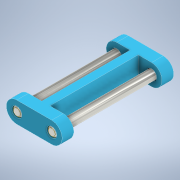
# Autodesk Inventor part: Lever
Saved by Autodesk Inventor 2021 (Build 250183000, 183)
## iProperties
Created: 2020-03-13
Part Number: Lever
Material: Generisch
Document SubType Name: Modeling
Designer: JochenAlt
Density: 1 g/cm^3
Appearance: Türkis
Author: JochenAlt
Autodesk Inventor part; units mm, degrees
ref_plane "YZ Plane" through (0, 0, 0) normal (1, 0, 0) x (0, 1, 0)
ref_plane "XZ Plane" through (0, 0, 0) normal (0, 1, 0) x (-1, 0, 0)
ref_plane "XY Plane" through (0, 0, 0) normal (0, 0, 1) x (1, 0, 0)
sketch "Skizze1" plane through (0, 0, 0) normal (0, 0, 1) x (1, 0, 0)
  line L0 (-12.15, 0) -> (4.65, 0) construction
  line L1 (0, -3.15) -> (0, 3.15) construction
  circle A0 centre (0, 0) radius 1.1
  circle A1 centre (-7.5, 0) radius 1.1
  line L2 (-7.5, 0) -> (0, 0) construction
  line L3 (-7.5, -2.25) -> (0, -2.25)
  line L4 (0, 2.25) -> (-7.5, 2.25)
  arc A2 (-7.5, 2.25) -> (-7.5, -2.25) centre (-7.5, 0) ccw
  arc A3 (0, -2.25) -> (0, 2.25) centre (0, 0) ccw
  line L5 (-4.625, 2.25) -> (-4.625, -2.25)
  line L6 (-2.875, 2.25) -> (-2.875, -2.25)
  line L7 (-3.75, 2.25) -> (-3.75, -2.25) construction
  circle A4 centre (-7.5, 0) radius 1
  circle A5 centre (0, 0) radius 1
  point P0 (-3.75, 0)
  dimension "d34" = 2.2
  dimension "d35" = 7.5
  dimension "d43" = 1.75
  dimension "d46" = 2
  dimension "d50" = 4.5
  constraints: 14 end point, 6 centre point, 5 point on line, 4 point on circle, 4 tangent, 3 midpoint, 2 coincident, 2 equal radius, 1 collinear, 1 parallel, 1 perpendicular, 1 vertical, 1 other
  measures "d34" diameter of A0
  measures "d35" distance of point (0, 0) L2.start
  measures "d43" distance between parallel lines of L6 L5
  measures "d46" diameter of A4
  measures "d50" distance between parallel lines of L3 L4
extrude "Extrusion9" add sketch "Skizze1" along normal mid plane 24 contours A2 L4 L5 L3 | L5 L4 L6 L3 | L6 L4 A3 L3
extrude "Extrusion10" cut sketch "Skizze1" along normal mid plane 19 contours A2 L4 L5 L3 | L5 L4 L6 L3 | L6 L4 A3 L3
extrude "Extrusion11" add sketch "Skizze1" along normal through all both and the other way through all contours L5 L4 L6 L3
extrude "Extrusion12" add sketch "Skizze1" along normal mid plane 24 separate body contours A4 | A5
chamfer "Fase1" distance 0.25 angle 45 4 edges at (-1, 0, 12) (-8.5, 0, 12) (-1, 0, -12) (-8.5, 0, -12)
